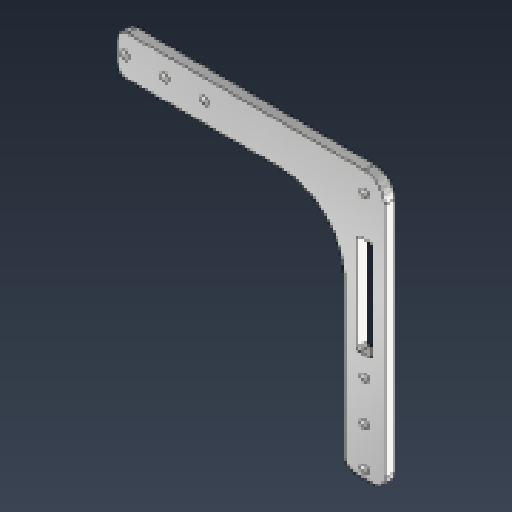
# Autodesk Inventor part: PLATE,CLAMP,MK4i,Swerve,CUSTOM,FRC2026
Saved by Autodesk Inventor 2026 (Build 300175050, 175E)
## iProperties
Created: 2021-12-05
Part Number: PLATE,CLAMP,MK4i,Swerve,CUSTOM,FRC2026
Material: Aluminum 7075
Document SubType Name: Modeling
Designer: dave.simone
Density: 2.81 g/cm^3
Appearance: Aluminum - Polished
Mass: 135.517 g
Surface Area: 208.301 cm^2
Volume: 48.2266 cm^3
Author: dave.simone
Revision Number: ANY
Autodesk Inventor part; units mm, degrees
ref_plane "Work Plane2" through (0, 0, 0) normal (-0.7071, 0.7071, 0) x (0, 0, 1)
ref_plane "XY Plane" through (0, 0, 0) normal (0, 0, 1) x (1, 0, 0)
ref_plane "Work Plane2" through (0, 0, 0) normal (-0.7071, 0.7071, 0) x (0, 0, 1)
sketch "Sketch1" plane through (-160.3375, 44.45, 0) normal (0, 0, 1) x (1, 0, 0)
  line L0 (311.15, -57.15) -> (160.3375, -57.15)
  arc A0 (311.15, -57.15) -> (317.5, -50.8) centre (311.15, -50.8) ccw
  line L1 (317.5, -38.1) -> (317.5, -50.8)
  arc A1 (317.5, -38.1) -> (311.15, -31.75) centre (311.15, -38.1) ccw
  line L2 (214.3125, -31.75) -> (311.15, -31.75)
  line L3 (173.0375, 106.3625) -> (173.0375, 9.525)
  arc A2 (173.0375, 106.3625) -> (166.6875, 112.7125) centre (166.6875, 106.3625) ccw
  line L4 (153.9875, 112.7125) -> (166.6875, 112.7125)
  arc A3 (153.9875, 112.7125) -> (147.6375, 106.3625) centre (153.9875, 106.3625) ccw
  line L5 (147.6375, -44.45) -> (147.6375, 106.3625)
  arc A4 (147.6375, -44.45) -> (160.3375, -57.15) centre (160.3375, -44.45) ccw
  line L6 (160.3375, -94.5418) -> (160.3375, 148.7892) construction
  line L7 (110.2457, -44.45) -> (353.5767, -44.45) construction
  arc A5 (173.0375, 9.525) -> (214.3125, -31.75) centre (214.3125, 9.525) ccw
  dimension "d1" = 169.8625
  dimension "d2" = 12.7
  dimension "d5" = 25.4
  dimension "d6" = 25.4
  dimension "d8" = 6.35
  dimension "d44" = 41.275
  constraints: 12 end point, 12 point on circle, 12 tangent, 6 centre point, 3 equal radius, 3 perpendicular, 2 parallel, 1 horizontal
  measures "d1" distance between parallel lines of L1 L5
  measures "d2" radius of A4
  measures "d5" distance between parallel lines of L2 L0
  measures "d6" distance between parallel lines of L5 L3
  measures "d8" radius of A0
  measures "d44" radius of A5
extrude "Extrusion1" add sketch "Sketch1" along normal mid plane 6.35
sketch "Sketch2" plane through (-160.3375, 44.45, 3.175) normal (0, 0, 1) x (1, 0, 0)
  line L0 (160.3375, -91.1225) -> (160.3375, 146.685) construction
  line L1 (113.665, -44.45) -> (351.4725, -44.45) construction
  line L2 (317.5, -50.8) -> (317.5, -38.1) construction
  point P0 (160.3375, -44.45)
  point P1 (312.7375, -44.45)
  dimension "d13" = 152.4
  constraints: 1 point on line
  measures "d13" distance from line of L0 point (312.738, -44.45)
hole "Hole1" at (152.4, 0, 3.175) direction (0, 0, -1) diameter 5.1054 end through all clearance for "Socket Head Cap Screw" size "#10" standard "Ansi Unified Screw Threads"
pattern_linear "Rectangular Pattern1" count 3 spacing 25.4 along (-1, 0, 0) of "Hole1"
sketch "Sketch4" plane through (-160.3375, 44.45, 3.175) normal (0, 0, 1) x (1, 0, 0)
  point P0 (160.3375, -44.45)
  point P1 (160.3375, -44.45)
  constraints: 1 coincident
hole "Hole2" at (0, 0, 3.175) direction (0, 0, -1) diameter 5.1054 end through all clearance for "Socket Head Cap Screw" size "#10" standard "Ansi Unified Screw Threads"
mirror "Mirror1" about plane through (0, 0, 0) normal (-0.7071, 0.7071, 0) of "Hole1", "Rectangular Pattern1"
sketch "Sketch5" plane through (-160.3375, 44.45, 3.175) normal (0, 0, 1) x (1, 0, 0)
  line L0 (163.5125, 38.1) -> (157.1625, 38.1)
  line L1 (155.575, 36.5125) -> (155.575, -17.4625)
  line L2 (157.1625, -19.05) -> (163.5125, -19.05)
  line L3 (165.1, -17.4625) -> (165.1, 36.5125)
  line L4 (160.3375, -91.1225) -> (160.3375, 146.685) construction
  arc A0 (165.1, 36.5125) -> (163.5125, 38.1) centre (163.5125, 36.5125) ccw
  arc A1 (157.1625, 38.1) -> (155.575, 36.5125) centre (157.1625, 36.5125) ccw
  arc A2 (155.575, -17.4625) -> (157.1625, -19.05) centre (157.1625, -17.4625) ccw
  arc A3 (163.5125, -19.05) -> (165.1, -17.4625) centre (163.5125, -17.4625) ccw
  point P0 (160.3375, -44.45)
  point P1 (155.575, -19.05)
  point P2 (155.575, 38.1)
  point P3 (165.1, -19.05)
  dimension "d45" = 9.525
  dimension "d46" = 25.4
  dimension "d47" = 57.15
  dimension "d48" = 1.5875
  constraints: 8 end point, 8 point on circle, 8 tangent, 6 point on line, 4 centre point, 3 equal radius, 2 parallel, 1 horizontal, 1 perpendicular, 1 other
  measures "d45" distance of point (155.575, -19.05) point (165.1, -19.05)
  measures "d46" distance from line of point (160.338, -44.45) L2
  measures "d47" distance of point (155.575, 38.1) point (155.575, -19.05)
  measures "d48" radius of A0
extrude "Extrusion3" cut sketch "Sketch5" against normal up to surface (6.35 mm away)
body "Solid18"
